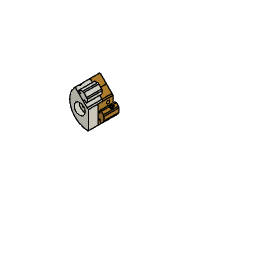
HINGE PART (Autodesk Fusion 360 design; units mm, degrees)
Autodesk Fusion 360 part; units mm, degrees
note: some values were not read from the file. Chosen so that the rebuilt part matches the saved one: which face or edge a step refers to. Set by a fixed rule: which sketch regions a step uses.
sketch "Sketch1" plane through (6.6339, 0, -6.5992) normal (0, -1, 0) x (1, 0, 0)
  circle A0 centre (10, 10) radius 2.5
  arc A1 (18.5, 0) -> (20, 1.5) centre (18.5, 1.5) ccw
  line L0 (20, 1.5) -> (20, 6.9)
  line L1 (20, 6.9) -> (18.2, 6.9)
  line L2 (18.2, 6.9) -> (18.2, 4.5)
  line L3 (18.2, 4.5) -> (16.5607, 4.5)
  line L4 (16.5607, 4.5) -> (14.4858, 6.5749)
  arc A2 (13.9, 7.9891) -> (14.4858, 6.5749) centre (15.9, 7.9891) ccw
  line L5 (13.9, 7.9891) -> (13.9, 12.0109)
  arc A3 (14.4858, 13.4251) -> (13.9, 12.0109) centre (15.9, 12.0109) ccw
  line L6 (14.4858, 13.4251) -> (16.5607, 15.5)
  line L7 (16.5607, 15.5) -> (18.2, 15.5)
  line L8 (18.2, 15.5) -> (18.2, 13.1)
  line L9 (18.2, 13.1) -> (20, 13.1)
  line L10 (20, 13.1) -> (20, 18.5)
  arc A4 (20, 18.5) -> (18.5, 20) centre (18.5, 18.5) ccw
  line L11 (18.5, 20) -> (13.1, 20)
  line L12 (13.1, 20) -> (13.1, 18.2)
  line L13 (13.1, 18.2) -> (15.5, 18.2)
  line L14 (15.5, 18.2) -> (15.5, 16.5607)
  line L15 (15.5, 16.5607) -> (13.4251, 14.4858)
  arc A5 (12.0109, 13.9) -> (13.4251, 14.4858) centre (12.0109, 15.9) ccw
  line L16 (12.0109, 13.9) -> (7.9891, 13.9)
  arc A6 (6.5749, 14.4858) -> (7.9891, 13.9) centre (7.9891, 15.9) ccw
  line L17 (6.5749, 14.4858) -> (4.5, 16.5607)
  line L18 (4.5, 16.5607) -> (4.5, 18.2)
  line L19 (4.5, 18.2) -> (6.9, 18.2)
  line L20 (6.9, 18.2) -> (6.9, 20)
  line L21 (6.9, 20) -> (1.5, 20)
  arc A7 (1.5, 20) -> (0, 18.5) centre (1.5, 18.5) ccw
  line L22 (0, 18.5) -> (0, 13.1)
  line L23 (0, 13.1) -> (1.8, 13.1)
  line L24 (1.8, 13.1) -> (1.8, 15.5)
  line L25 (1.8, 15.5) -> (3.4393, 15.5)
  line L26 (3.4393, 15.5) -> (5.5142, 13.4251)
  arc A8 (6.1, 12.0109) -> (5.5142, 13.4251) centre (4.1, 12.0109) ccw
  line L27 (6.1, 12.0109) -> (6.1, 7.9891)
  arc A9 (5.5142, 6.5749) -> (6.1, 7.9891) centre (4.1, 7.9891) ccw
  line L28 (5.5142, 6.5749) -> (3.4393, 4.5)
  line L29 (3.4393, 4.5) -> (1.8, 4.5)
  line L30 (1.8, 4.5) -> (1.8, 6.9)
  line L31 (1.8, 6.9) -> (0, 6.9)
  line L32 (0, 6.9) -> (0, 1.5)
  arc A10 (0, 1.5) -> (1.5, 0) centre (1.5, 1.5) ccw
  line L33 (1.5, 0) -> (6.9, 0)
  line L34 (6.9, 0) -> (6.9, 1.8)
  line L35 (6.9, 1.8) -> (4.5, 1.8)
  line L36 (4.5, 1.8) -> (4.5, 3.4393)
  line L37 (4.5, 3.4393) -> (6.5749, 5.5142)
  arc A11 (7.9891, 6.1) -> (6.5749, 5.5142) centre (7.9891, 4.1) ccw
  line L38 (7.9891, 6.1) -> (12.0109, 6.1)
  arc A12 (13.4251, 5.5142) -> (12.0109, 6.1) centre (12.0109, 4.1) ccw
  line L39 (13.4251, 5.5142) -> (15.5, 3.4393)
  line L40 (15.5, 3.4393) -> (15.5, 1.8)
  line L41 (15.5, 1.8) -> (13.1, 1.8)
  line L42 (13.1, 1.8) -> (13.1, 0)
  line L43 (13.1, 0) -> (18.5, 0)
  line L44 (0, 18.5) -> (0, 20)
  line L45 (0, 20) -> (1.5, 20)
  line L46 (3.6062, 26.1518) -> (1.9092, 24.4548)
  line L47 (-4.879, 43.4052) -> (-3.6062, 42.1324)
  arc A13 (-0.75, 28.5483) -> (-1.3358, 29.9625) centre (-2.75, 28.5483) ccw
  line L48 (4.1796, 35.4779) -> (1.3358, 38.3218)
  arc A14 (-1.0607, 21.0607) -> (1.0607, 21.0607) centre (0, 22.1213) ccw
  circle A15 centre (0, 34.1421) radius 2.5
  line L49 (-4.1796, 32.8063) -> (-1.3358, 29.9625)
  arc A16 (-1.3358, 38.3218) -> (-0.75, 39.736) centre (-2.75, 39.736) ccw
  line L50 (-7.9903, 37.7484) -> (-9.2631, 39.0212)
  line L51 (0.75, 25.614) -> (0.75, 28.5483)
  line L52 (1.0607, 21.0607) -> (4.879, 24.879)
  line L53 (-1.9092, 24.4548) -> (-3.6062, 26.1518)
  line L54 (-3.6062, 42.1324) -> (-1.9092, 43.8295)
  arc A17 (4.1796, 35.4779) -> (5.5939, 34.8921) centre (5.5939, 36.8921) ccw
  line L55 (0, 20) -> (-1.0607, 21.0607)
  line L56 (-0.75, 25.614) -> (-1.9092, 24.4548)
  line L57 (8.5282, 34.8921) -> (5.5939, 34.8921)
  arc A18 (0.75, 39.736) -> (1.3358, 38.3218) centre (2.75, 39.736) ccw
  arc A19 (13.0815, 33.0815) -> (13.0815, 35.2028) centre (12.0208, 34.1421) ccw
  line L58 (8.5282, 33.3921) -> (9.6874, 32.2329)
  line L59 (4.879, 24.879) -> (3.6062, 26.1518)
  line L60 (-5.5939, 34.8921) -> (-8.5282, 34.8921)
  line L61 (-1.3358, 38.3218) -> (-4.1796, 35.4779)
  line L62 (-7.9903, 30.5359) -> (-9.6874, 32.2329)
  arc A20 (-5.5939, 34.8921) -> (-4.1796, 35.4779) centre (-5.5939, 36.8921) ccw
  line L63 (-9.6874, 36.0513) -> (-7.9903, 37.7484)
  arc A21 (-4.1796, 32.8063) -> (-5.5939, 33.3921) centre (-5.5939, 31.3921) ccw
  arc A22 (-13.0815, 35.2028) -> (-13.0815, 33.0815) centre (-12.0208, 34.1421) ccw
  line L64 (-9.2631, 29.2631) -> (-7.9903, 30.5359)
  line L65 (-1.0607, 47.2236) -> (-4.879, 43.4052)
  line L66 (-13.0815, 33.0815) -> (-9.2631, 29.2631)
  line L67 (13.0815, 35.2028) -> (9.2631, 39.0212)
  line L68 (9.2631, 29.2631) -> (13.0815, 33.0815)
  arc A23 (5.5939, 33.3921) -> (4.1796, 32.8063) centre (5.5939, 31.3921) ccw
  line L69 (1.9092, 43.8295) -> (3.6062, 42.1324)
  line L70 (1.9092, 24.4548) -> (0.75, 25.614)
  line L71 (7.9903, 30.5359) -> (9.2631, 29.2631)
  line L72 (-3.6062, 26.1518) -> (-4.879, 24.879)
  line L73 (-9.6874, 32.2329) -> (-8.5282, 33.3921)
  line L74 (7.9903, 37.7484) -> (9.6874, 36.0513)
  line L75 (9.6874, 36.0513) -> (8.5282, 34.8921)
  line L76 (-8.5282, 34.8921) -> (-9.6874, 36.0513)
  line L77 (1.3358, 29.9625) -> (4.1796, 32.8063)
  line L78 (-9.2631, 39.0212) -> (-13.0815, 35.2028)
  line L79 (4.879, 43.4052) -> (1.0607, 47.2236)
  line L80 (9.6874, 32.2329) -> (7.9903, 30.5359)
  line L81 (-8.5282, 33.3921) -> (-5.5939, 33.3921)
  line L82 (-4.879, 24.879) -> (-1.0607, 21.0607)
  line L83 (-1.9092, 43.8295) -> (-0.75, 42.6703)
  line L84 (0.75, 39.736) -> (0.75, 42.6703)
  line L85 (-0.75, 28.5483) -> (-0.75, 25.614)
  line L86 (3.6062, 42.1324) -> (4.879, 43.4052)
  arc A24 (1.3358, 29.9625) -> (0.75, 28.5483) centre (2.75, 28.5483) ccw
  line L87 (1.0607, 21.0607) -> (0, 20)
  line L88 (0.75, 42.6703) -> (1.9092, 43.8295)
  arc A25 (1.0607, 47.2236) -> (-1.0607, 47.2236) centre (0, 46.163) ccw
  line L89 (5.5939, 33.3921) -> (8.5282, 33.3921)
  line L90 (-0.75, 42.6703) -> (-0.75, 39.736)
  line L91 (9.2631, 39.0212) -> (7.9903, 37.7484)
  arc A26 (-13.0815, 33.0815) -> (0, 1.5) centre (0, 20) ccw
  point P0 (14.1421, 34.1421)
  constraint coincident A7.end L22.start
  constraint tangent A7 L44
  constraint coincident L21.end A7.start
  constraint tangent A7 L45
  constraint coincident A14.end L52.start
  constraint tangent A14 L87
  constraint coincident A14.start L55.end
  constraint tangent A14 L55
  constraint coincident L44.end L45.start
extrude "Extrude1" add sketch "Sketch1" along normal blind 5 contours L22 L23 L24 L25 L26 A8 L27 A9 L28 L29 L30 L31 L32 L44 A13 L49 L53 L55 L56 L62 A21 L64 L66 L72 L73 L81 L82 L85 A26 makes body 1
sketch "Sketch2" plane through (0, -5, 0) normal (0, -1, 0) x (1, 0, 0)
  line L0 (-2.6292, 22.6639) -> (-6.4476, 26.4823)
  arc A0 (-6.4476, 26.4823) -> (6.6339, -5.0992) centre (6.6339, 13.4008) ccw
  line L1 (6.6339, -5.0992) -> (6.6339, 0.3008)
  line L2 (6.6339, 0.3008) -> (8.4339, 0.3008)
  line L3 (8.4339, 0.3008) -> (8.4339, -2.0992)
  line L4 (8.4339, -2.0992) -> (10.0732, -2.0992)
  line L5 (10.0732, -2.0992) -> (12.1481, -0.0243)
  arc A1 (12.1481, -0.0243) -> (12.7339, 1.3899) centre (10.7339, 1.3899) ccw
  line L6 (12.7339, 1.3899) -> (12.7339, 5.4117)
  arc A2 (12.7339, 5.4117) -> (12.1481, 6.8259) centre (10.7339, 5.4117) ccw
  line L7 (12.1481, 6.8259) -> (10.0732, 8.9008)
  line L8 (10.0732, 8.9008) -> (8.4339, 8.9008)
  line L9 (8.4339, 8.9008) -> (8.4339, 6.5008)
  line L10 (8.4339, 6.5008) -> (6.6339, 6.5008)
  line L11 (6.6339, 6.5008) -> (6.6339, 13.4008)
  line L12 (6.6339, 13.4008) -> (5.5732, 14.4615)
  line L13 (5.5732, 14.4615) -> (1.7548, 18.2799)
  line L14 (1.7548, 18.2799) -> (3.0276, 19.5526)
  line L15 (3.0276, 19.5526) -> (4.7247, 17.8556)
  line L16 (4.7247, 17.8556) -> (5.8839, 19.0148)
  line L17 (5.8839, 19.0148) -> (5.8839, 21.9491)
  arc A3 (5.8839, 21.9491) -> (5.2981, 23.3633) centre (3.8839, 21.9491) ccw
  line L18 (5.2981, 23.3633) -> (2.4542, 26.2072)
  arc A4 (2.4542, 26.2072) -> (1.04, 26.793) centre (1.04, 24.793) ccw
  line L19 (1.04, 26.793) -> (-1.8943, 26.793)
  line L20 (-1.8943, 26.793) -> (-3.0535, 25.6338)
  line L21 (-3.0535, 25.6338) -> (-1.3564, 23.9367)
  line L22 (-1.3564, 23.9367) -> (-2.6292, 22.6639)
  line L23 (6.6339, 13.4008) -> (-11.8661, 13.4008)
  constraint coincident A0.centre L11.end
  constraint coincident A0 L23.end
  constraint perpendicular L11 L23
extrude "Extrude2" add sketch "Sketch2" along normal blind 5 contours A0 L1 L2 L3 L4 L5 A1 L6 A2 L7 L8 L9 L10 L11 L23 bodies 1
extrude "Extrude3" add 1 faces at (-4.0367, -5, 19.7109) along direction (0, -1, 0) blind 5 on bodies 1 bodies 1
extrude "Extrude4" add 1 faces at (0.6709, -10, 8.8926) along direction (0, -1, 0) blind 10 on bodies 1 bodies 1
ref_plane "WorkPlane1" through (-1.2272, -10, 10.8469) normal (0, -1, 0) x (1, 0, 0)
sketch "Sketch3" plane through (-7.8611, -10, 17.4461) normal (0, -1, 0) x (1, 0, 0)
  arc A0 (1.4135, 9.0362) -> (14.495, -22.5452) centre (14.495, -4.0452) ccw
  line L0 (14.495, -22.5452) -> (14.495, -17.1452)
  line L1 (14.495, -17.1452) -> (16.295, -17.1452)
  line L2 (16.295, -17.1452) -> (16.295, -19.5452)
  line L3 (16.295, -19.5452) -> (17.9343, -19.5452)
  line L4 (17.9343, -19.5452) -> (20.0092, -17.4704)
  arc A1 (20.0092, -17.4704) -> (20.595, -16.0562) centre (18.595, -16.0562) ccw
  line L5 (20.595, -16.0562) -> (20.595, -12.0343)
  arc A2 (20.595, -12.0343) -> (20.0092, -10.6201) centre (18.595, -12.0343) ccw
  line L6 (20.0092, -10.6201) -> (17.9343, -8.5452)
  line L7 (17.9343, -8.5452) -> (16.295, -8.5452)
  line L8 (16.295, -8.5452) -> (16.295, -10.9452)
  line L9 (16.295, -10.9452) -> (14.495, -10.9452)
  line L10 (14.495, -10.9452) -> (14.495, -4.0452)
  line L11 (14.495, -4.0452) -> (13.4343, -2.9846)
  line L12 (13.4343, -2.9846) -> (9.616, 0.8338)
  line L13 (9.616, 0.8338) -> (10.8887, 2.1066)
  line L14 (10.8887, 2.1066) -> (12.5858, 0.4095)
  line L15 (12.5858, 0.4095) -> (13.745, 1.5687)
  line L16 (13.745, 1.5687) -> (13.745, 4.503)
  arc A3 (13.745, 4.503) -> (13.1592, 5.9172) centre (11.745, 4.503) ccw
  line L17 (13.1592, 5.9172) -> (10.3153, 8.7611)
  arc A4 (10.3153, 8.7611) -> (8.9011, 9.3469) centre (8.9011, 7.3469) ccw
  line L18 (8.9011, 9.3469) -> (5.9668, 9.3469)
  line L19 (5.9668, 9.3469) -> (4.8076, 8.1877)
  line L20 (4.8076, 8.1877) -> (6.5047, 6.4906)
  line L21 (6.5047, 6.4906) -> (5.2319, 5.2179)
  line L22 (5.2319, 5.2179) -> (1.4135, 9.0362)
  line L23 (14.495, -4.0452) -> (1.4135, -17.1267)
  line L24 (14.495, -4.0452) -> (32.995, -4.0452) construction
  dimension "d12" = 135
  constraint horizontal L24
  constraint coincident A0.centre L10.end
  constraint coincident A0 L23.end
  measures "d12" angle of L23 L24
extrude "Extrude5" cut 1 faces at (0.6709, -20, 8.8926) along direction (0, 1, 0) blind 10 on bodies 1 bodies 1
extrude "Extrude6" cut sketch "Sketch3" against normal blind 5 contours A0 L11 L12 L13 L14 L15 L16 A3 L17 A4 L18 L19 L20 L21 L22 L23 bodies 1
extrude "Extrude7" add 1 faces at (-1.0433, -5, 13.0208) along direction (0, -1, 0) blind 10 separate body on bodies 1 makes body 2
extrude "Extrude8" add 1 faces at (2.2734, -10, 6.7403) along direction (0, -1, 0) blind 5 separate body on bodies 1 makes body 3
combine "Combine1" operation add target body 3 tool bodies 2
sketch "Sketch4" plane through (0, -15, 0) normal (0, -1, 0) x (1, 0, 0)
  arc A0 (-6.4476, 26.4823) -> (6.6339, -5.0992) centre (6.6339, 13.4008) ccw
  line L0 (6.6339, -5.0992) -> (6.6339, 0.3008)
  line L1 (6.6339, 0.3008) -> (8.4339, 0.3008)
  line L2 (8.4339, 0.3008) -> (8.4339, -2.0992)
  line L3 (8.4339, -2.0992) -> (10.0732, -2.0992)
  line L4 (10.0732, -2.0992) -> (12.1481, -0.0243)
  arc A1 (12.1481, -0.0243) -> (12.7339, 1.3899) centre (10.7339, 1.3899) ccw
  line L5 (12.7339, 1.3899) -> (12.7339, 5.4117)
  arc A2 (12.7339, 5.4117) -> (12.1481, 6.8259) centre (10.7339, 5.4117) ccw
  line L6 (12.1481, 6.8259) -> (10.0732, 8.9008)
  line L7 (10.0732, 8.9008) -> (8.4339, 8.9008)
  line L8 (8.4339, 8.9008) -> (8.4339, 6.5008)
  line L9 (8.4339, 6.5008) -> (6.6339, 6.5008)
  line L10 (6.6339, 6.5008) -> (6.6339, 13.4008)
  line L11 (6.6339, 13.4008) -> (5.5732, 14.4615)
  line L12 (5.5732, 14.4615) -> (1.7548, 18.2799)
  line L13 (1.7548, 18.2799) -> (3.0276, 19.5526)
  line L14 (3.0276, 19.5526) -> (4.7247, 17.8556)
  line L15 (4.7247, 17.8556) -> (5.8839, 19.0148)
  line L16 (5.8839, 19.0148) -> (5.8839, 21.9491)
  arc A3 (5.8839, 21.9491) -> (5.2981, 23.3633) centre (3.8839, 21.9491) ccw
  line L17 (5.2981, 23.3633) -> (2.4542, 26.2072)
  arc A4 (2.4542, 26.2072) -> (1.04, 26.793) centre (1.04, 24.793) ccw
  line L18 (1.04, 26.793) -> (-1.8943, 26.793)
  line L19 (-1.8943, 26.793) -> (-3.0535, 25.6338)
  line L20 (-3.0535, 25.6338) -> (-1.3564, 23.9367)
  line L21 (-1.3564, 23.9367) -> (-2.6292, 22.6639)
  line L22 (-2.6292, 22.6639) -> (-6.4476, 26.4823)
  line L23 (6.6339, 13.4008) -> (-10.4579, 6.3212)
  circle A5 centre (-1.912, 9.861) radius 2.5
  circle A6 centre (-1.912, 9.861) radius 5
  dimension "d21" = 5
  dimension "d24" = 10
  constraint coincident A0.centre L10.end
  constraint midpoint A0 L23.end
  constraint midpoint L23 A5.centre
  constraint concentric A5 A6
  measures "d21" diameter of A5
  measures "d24" diameter of A6
extrude "Extrude9" cut sketch "Sketch4" against normal blind 17 contours L23 A5 | L23 A5 bodies 1 3
extrude "Extrude10" add 1 faces at (-5.5635, -15, 17.6804) along direction (0, -1, 0) blind 5 on bodies 3 bodies 3
extrude "Extrude11" add 1 faces at (1.4531, 0, 1.5039) along direction (0, 1, 0) blind 5 on bodies 1 bodies 1
sketch "Sketch5" plane through (0, -20, 0) normal (0, -1, 0) x (1, 0, 0)
  circle A0 centre (-1.912, 9.861) radius 2.5
  arc A1 (-6.4476, 26.4823) -> (6.6339, -5.0992) centre (6.6339, 13.4008) ccw
  line L0 (6.6339, -5.0992) -> (6.6339, 0.3008)
  line L1 (6.6339, 0.3008) -> (8.4339, 0.3008)
  line L2 (8.4339, 0.3008) -> (8.4339, -2.0992)
  line L3 (8.4339, -2.0992) -> (10.0732, -2.0992)
  line L4 (10.0732, -2.0992) -> (12.1481, -0.0243)
  arc A2 (12.1481, -0.0243) -> (12.7339, 1.3899) centre (10.7339, 1.3899) ccw
  line L5 (12.7339, 1.3899) -> (12.7339, 5.4117)
  arc A3 (12.7339, 5.4117) -> (12.1481, 6.8259) centre (10.7339, 5.4117) ccw
  line L6 (12.1481, 6.8259) -> (10.0732, 8.9008)
  line L7 (10.0732, 8.9008) -> (8.4339, 8.9008)
  line L8 (8.4339, 8.9008) -> (8.4339, 6.5008)
  line L9 (8.4339, 6.5008) -> (6.6339, 6.5008)
  line L10 (6.6339, 6.5008) -> (6.6339, 13.4008)
  line L11 (6.6339, 13.4008) -> (5.5732, 14.4615)
  line L12 (5.5732, 14.4615) -> (1.7548, 18.2799)
  line L13 (1.7548, 18.2799) -> (3.0276, 19.5526)
  line L14 (3.0276, 19.5526) -> (4.7247, 17.8556)
  line L15 (4.7247, 17.8556) -> (5.8839, 19.0148)
  line L16 (5.8839, 19.0148) -> (5.8839, 21.9491)
  arc A4 (5.8839, 21.9491) -> (5.2981, 23.3633) centre (3.8839, 21.9491) ccw
  line L17 (5.2981, 23.3633) -> (2.4542, 26.2072)
  arc A5 (2.4542, 26.2072) -> (1.04, 26.793) centre (1.04, 24.793) ccw
  line L18 (1.04, 26.793) -> (-1.8943, 26.793)
  line L19 (-1.8943, 26.793) -> (-3.0535, 25.6338)
  line L20 (-3.0535, 25.6338) -> (-1.3564, 23.9367)
  line L21 (-1.3564, 23.9367) -> (-2.6292, 22.6639)
  line L22 (-2.6292, 22.6639) -> (-6.4476, 26.4823)
  circle A6 centre (-1.912, 9.861) radius 2.5
  circle A7 centre (-1.912, 9.861) radius 5.5
  line L23 (6.6339, 0.3008) -> (6.6339, 6.5008)
  dimension "d29" = 11
  constraint concentric A0 A7
  constraint coincident L0.end L1.start
  constraint coincident L9.end L10.start
  measures "d29" diameter of A7
extrude "Extrude12" cut sketch "Sketch5" against normal blind 5 contours A7 bodies 3
sketch "Sketch6" plane through (0, 5, 0) normal (0, 1, 0) x (-1, 0, 0)
  circle A0 centre (1.912, 9.861) radius 2.5
  line L0 (6.4476, 26.4823) -> (2.6292, 22.6639)
  line L1 (2.6292, 22.6639) -> (1.3564, 23.9367)
  line L2 (1.3564, 23.9367) -> (3.0535, 25.6338)
  line L3 (3.0535, 25.6338) -> (1.8943, 26.793)
  line L4 (1.8943, 26.793) -> (-1.04, 26.793)
  arc A1 (-1.04, 26.793) -> (-2.4542, 26.2072) centre (-1.04, 24.793) ccw
  line L5 (-2.4542, 26.2072) -> (-5.2981, 23.3633)
  arc A2 (-5.2981, 23.3633) -> (-5.8839, 21.9491) centre (-3.8839, 21.9491) ccw
  line L6 (-5.8839, 21.9491) -> (-5.8839, 19.0148)
  line L7 (-5.8839, 19.0148) -> (-4.7247, 17.8556)
  line L8 (-4.7247, 17.8556) -> (-3.0276, 19.5526)
  line L9 (-3.0276, 19.5526) -> (-1.7548, 18.2799)
  line L10 (-1.7548, 18.2799) -> (-5.5732, 14.4615)
  line L11 (-5.5732, 14.4615) -> (-6.6339, 13.4008)
  line L12 (-6.6339, 13.4008) -> (-6.6339, 6.5008)
  line L13 (-6.6339, 6.5008) -> (-8.4339, 6.5008)
  line L14 (-8.4339, 6.5008) -> (-8.4339, 8.9008)
  line L15 (-8.4339, 8.9008) -> (-10.0732, 8.9008)
  line L16 (-10.0732, 8.9008) -> (-12.1481, 6.8259)
  arc A3 (-12.1481, 6.8259) -> (-12.7339, 5.4117) centre (-10.7339, 5.4117) ccw
  line L17 (-12.7339, 5.4117) -> (-12.7339, 1.3899)
  arc A4 (-12.7339, 1.3899) -> (-12.1481, -0.0243) centre (-10.7339, 1.3899) ccw
  line L18 (-12.1481, -0.0243) -> (-10.0732, -2.0992)
  line L19 (-10.0732, -2.0992) -> (-8.4339, -2.0992)
  line L20 (-8.4339, -2.0992) -> (-8.4339, 0.3008)
  line L21 (-8.4339, 0.3008) -> (-6.6339, 0.3008)
  line L22 (-6.6339, 0.3008) -> (-6.6339, -5.0992)
  arc A5 (-6.6339, -5.0992) -> (6.4476, 26.4823) centre (-6.6339, 13.4008) ccw
  line L23 (-2.7068, 9.861) -> (-0.3974, 5.861)
  line L24 (-0.3974, 5.861) -> (4.2214, 5.861)
  line L25 (4.2214, 5.861) -> (6.5308, 9.861)
  line L26 (6.5308, 9.861) -> (4.2214, 13.861)
  line L27 (4.2214, 13.861) -> (-0.3974, 13.861)
  line L28 (-0.3974, 13.861) -> (-2.7068, 9.861)
  line L29 (2.6292, 22.6639) -> (-1.7548, 18.2799)
  point P0 (1.912, 9.861)
  dimension "d32" = 4
  constraint coincident P0 A0.centre
  constraint coincident L0.end L1.start
  constraint coincident L9.end L10.start
  constraint parallel L13 L24
  measures "d32" distance of P0 L28
extrude "Extrude13" cut sketch "Sketch6" against normal blind 5 contours L23 L24 L25 L26 L27 L28 bodies 1
extrude "Extrude14" cut sketch "Sketch6" against normal blind 10 contours L1 L2 L3 L4 A1 L5 A2 L6 L7 L8 L9 L29 bodies 1
extrude "Extrude15" cut sketch "Sketch5" against normal blind 10 contours L1 L2 L3 L4 A2 L5 A3 L6 L7 L8 L9 L23 bodies 3
move_face "OffsetFaces1" offset -0.25 20 faces at (12.7339, -5, 4.0711) (12.266, 0, 6.6973) (10.7648, -5, 8.2092) (7.8339, 0, 6.5008) (8.9803, -5, 8.9008) (8.4339, -5, -0.4992) (9.5268, -5, -2.0992) (11.4565, 0, -0.7159) (7.2339, 0, 0.3008) (12.7263, 0, 1.2156) (5.8839, -15, 19.9929) (5.8763, -15, 22.1234) (3.4022, -15, 25.2592) (2.3912, -15, 26.2675) (-0.9162, -15, 26.793) (-2.6671, -15, 26.0202) (-1.7807, -15, 23.5124) (2.6034, -15, 19.1284) (3.5933, -15, 18.987) (5.4975, -15, 18.6284) on bodies 1 3
sketch "Sketch11" plane through (12.4839, 0, 0) normal (1, 0, 0) x (0, 1, 0)
  line L0 (-10, 5.4117) -> (-10, 1.3899)
  line L1 (-10, 1.3899) -> (5, 1.3899)
  line L2 (5, 1.3899) -> (5, 5.4117)
  line L3 (5, 5.4117) -> (-10, 5.4117)
  line L4 (1.5588, 7.3117) -> (3.1177, 10.0117)
  line L5 (3.1177, 10.0117) -> (1.5588, 12.7117)
  line L6 (1.5588, 12.7117) -> (-1.5588, 12.7117)
  line L7 (-1.5588, 12.7117) -> (-3.1177, 10.0117)
  line L8 (-3.1177, 10.0117) -> (-1.5588, 7.3117)
  line L9 (-1.5588, 7.3117) -> (1.5588, 7.3117)
  line L10 (5, 5.4117) -> (5, 1.3899)
  point P0 (0, 10.0117)
  dimension "d68" = 2.7
  dimension "d69" = 5
  constraint parallel L1 L9
  measures "d68" distance of P0 L9
  measures "d69" distance of P0 L10
extrude "Extrude22" cut sketch "Sketch11" against normal blind 2.5 contours L4 L5 L6 L7 L8 L9 bodies 1
sketch "Sketch12" plane through (9.9839, 0, 0) normal (1, 0, 0) x (0, 1, 0)
  line L0 (-1.5588, 7.3117) -> (1.5588, 7.3117)
  line L1 (1.5588, 7.3117) -> (2.3238, 8.6366)
  line L2 (-2.3238, 8.6366) -> (-1.5588, 7.3117)
  circle A0 centre (0, 10) radius 1.5
  line L3 (2.3238, 8.6366) -> (-2.3238, 8.6366)
  dimension "d72" = 3
  measures "d72" diameter of A0
extrude "Extrude23" cut sketch "Sketch12" against normal blind 22 contours A0 L3 | A0 L3 bodies 1
ref_plane "WorkPlane2" through (-0.0161, 0, 7.9742) normal (1, 0, 0) x (0, 0, -1)
sketch "Sketch13" plane through (-0.0161, 0, 10.0117) normal (1, 0, 0) x (0, 1, 0)
  spline S0 degree 3 poles (0, -1.5117) (0.1884, -1.5117) (0.3888, -1.474) (0.7564, -1.3222) (0.9236, -1.2082) (1.1906, -0.9438) (1.3071, -0.7745) (1.4619, -0.4034) (1.5, -0.2015) (1.5, 0.1758) (1.4627, 0.3766) (1.3093, 0.7471) (1.1933, 0.9168) (0.9259, 1.1832) (0.7577, 1.2981) (0.3888, 1.4507) (0.1882, 1.4883) (-0.1882, 1.4883) (-0.3888, 1.4507) (-0.7577, 1.2981) (-0.9259, 1.1832) (-1.1933, 0.9168) (-1.3093, 0.7471) (-1.4627, 0.3766) (-1.5, 0.1758) (-1.5, -0.2015) (-1.4619, -0.4034) (-1.3071, -0.7745) (-1.1906, -0.9438) (-0.9236, -1.2082) (-0.7564, -1.3222) (-0.3888, -1.474) (-0.1884, -1.5117) (0, -1.5117) knots 0 0 0 0 0.05652 0.05652 0.11304 0.11304 0.170954 0.170954 0.228868 0.228868 0.286089 0.286089 0.343311 0.343311 0.399757 0.399757 0.456203 0.456203 0.512649 0.512649 0.569095 0.569095 0.626316 0.626316 0.683538 0.683538 0.741452 0.741452 0.799366 0.799366 0.855886 0.855886 0.912406 0.912406 0.912406 0.912406
  circle A0 centre (0, 0) radius 2.75
  point P0 (0, -1.5117)
  dimension "d76" = 5.5
  constraint coincident A0.centre origin
  measures "d76" diameter of A0
extrude "Extrude24" cut sketch "Sketch13" against normal blind 14 bodies 1
sketch "Sketch14" plane through (14.1539, 0, 14.1539) normal (0.707107, 0, 0.707107) x (0, 1, 0)
  line L0 (-5, 12.774) -> (-5, 16.7959)
  line L1 (-5, 16.7959) -> (-20, 16.7959)
  line L2 (-20, 16.7959) -> (-20, 12.774)
  line L3 (-20, 12.774) -> (-5, 12.774)
  line L4 (-13.4412, 21.3) -> (-11.8823, 24)
  line L5 (-11.8823, 24) -> (-13.4412, 26.7)
  line L6 (-13.4412, 26.7) -> (-16.5588, 26.7)
  line L7 (-16.5588, 26.7) -> (-18.1177, 24)
  line L8 (-18.1177, 24) -> (-16.5588, 21.3)
  line L9 (-16.5588, 21.3) -> (-13.4412, 21.3)
  line L10 (-5, 11.5366) -> (-20, 11.5366)
  point P0 (-15, 24)
  dimension "d79" = 2.7
  constraint parallel L9 L10
  measures "d79" distance of P0 L9
extrude "Extrude25" cut sketch "Sketch14" against normal blind 2.5 contours L4 L5 L6 L7 L8 L9 bodies 3
sketch "Sketch15" plane through (12.3688, 0, 12.3688) normal (0.707107, 0, 0.707107) x (0, 1, 0)
  line L0 (-16.5588, 21.3) -> (-13.4412, 21.3)
  line L1 (-13.4412, 21.3) -> (-11.8823, 24)
  line L2 (-11.8823, 24) -> (-13.4412, 26.7)
  line L3 (-13.4412, 26.7) -> (-16.5588, 26.7)
  line L4 (-16.5588, 26.7) -> (-18.1177, 24)
  line L5 (-18.1177, 24) -> (-16.5588, 21.3)
  circle A0 centre (-15, 24) radius 1.5
  dimension "d82" = 3
  measures "d82" diameter of A0
extrude "Extrude26" cut sketch "Sketch15" against normal blind 23 contours A0 bodies 3
ref_plane "WorkPlane3" through (-11.6728, -15, 22.2683) normal (0.707107, 0, 0.707107) x (0.707107, 0, -0.707107)
sketch "Sketch16" plane through (-11.6728, -15, 22.2683) normal (0.707107, 0, 0.707107) x (0.707107, 0, -0.707107)
  circle A0 centre (0, 0) radius 2.75
  dimension "d86" = 5.5
  constraint coincident A0.centre origin
  measures "d86" diameter of A0
extrude "Extrude27" cut sketch "Sketch16" against normal blind 12 bodies 3
split "Split1" by plane through (-2.6292, -15, 22.6639) normal (0.707107, 0, 0.707107) bodies 3 makes body 4 at (4.1734, -10, 24.1345)
split "Split2" by plane through (0, 0, 0) normal (1, 0, 0) bodies 1 makes body 5 at (2.3438, 5, 0.8477)
copy_body "Body->Comp1" bodies 5 removing the originals makes body 6 in component "Component"
copy_body "Body->Comp2" bodies 3 removing the originals makes body 7 in component "Component'"
copy_body "Body->Comp3" bodies 4 removing the originals makes body 8 in component "Component''"
copy_body "Body->Comp4" bodies 1 removing the originals makes body 9 in component "Component'''"
component "Component" placed x (1, 0, 0) y (0, 1, 0) z (0, 0, 1) at (0, 0, 0)
component "Component'" placed x (1, 0, 0) y (0, 1, 0) z (0, 0, 1) at (0, 0, 0)
component "Component''" placed x (1, 0, 0) y (0, 1, 0) z (0, 0, 1) at (0, 0, 0)
component "Component'''" placed x (1, 0, 0) y (0, 1, 0) z (0, 0, 1) at (0, 0, 0)
